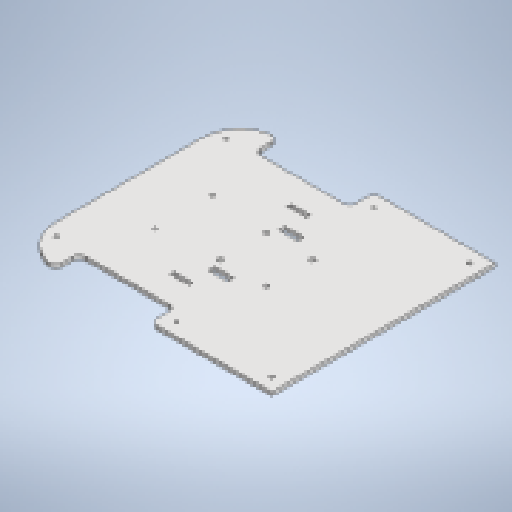
# Autodesk Inventor part: Base_Carro
Saved by Autodesk Inventor 2024 (Build 280153000, 153)
## iProperties
Created: 2025-05-13
Part Number: Base_Carro
Material: Genérico
Document SubType Name: Modeling
Designer: mario
Density: 1 g/cm^3
Appearance: Valor por defecto
Author: mario
Autodesk Inventor part; units mm, degrees
ref_plane "YZ Plane" through (0, 0, 0) normal (1, 0, 0) x (0, 1, 0)
ref_plane "XZ Plane" through (0, 0, 0) normal (0, 1, 0) x (-1, 0, 0)
ref_plane "XY Plane" through (0, 0, 0) normal (0, 0, 1) x (1, 0, 0)
sketch "Boceto1" plane through (0, 0, 0) normal (0, 1, 0) x (-1, 0, 0)
  line L0 (100, 87.5) -> (-100, 87.5)
  line L1 (-100, 87.5) -> (-100, -87.5)
  line L2 (-100, -87.5) -> (100, -87.5)
  line L3 (100, -87.5) -> (100, 87.5)
  line L4 (100, 87.5) -> (-100, -87.5) construction
  line L5 (-100, 87.5) -> (100, -87.5) construction
  point P0 (0, 0)
  dimension "d0" = 175
  dimension "d1" = 200
  constraints: 12 end point, 2 midpoint, 2 parallel, 1 horizontal, 1 perpendicular
  measures "d0" distance of L2.end L0.start
  measures "d1" distance of L1.end L2.end
extrude "Extrusión1" add sketch "Boceto1" along normal blind 3
sketch "Boceto2" plane through (0, 3, 0) normal (0, 1, 0) x (1, 0, 0)
  line L0 (-4.8, 47.5) -> (-20, 47.5)
  line L1 (-20, 47.5) -> (-20, 44.4)
  line L2 (-20, 44.4) -> (-4.8, 44.4)
  line L3 (-4.8, 44.4) -> (-4.8, 47.5)
  line L4 (100, 87.5) -> (-100, 87.5) construction
  line L5 (-100, 87.5) -> (-100, -87.5) construction
  point P0 (0, 0)
  dimension "d4" = 15.2
  dimension "d5" = 3.1
  dimension "d6" = 40
  dimension "d7" = 80
  constraints: 8 end point, 2 parallel, 1 horizontal, 1 perpendicular
  measures "d4" distance of L2.end L1.end
  measures "d5" distance of L2.end L0.start
  measures "d6" distance between parallel lines of L4 L0
  measures "d7" distance between parallel lines of L5 L1
extrude "Extrusión2" cut sketch "Boceto2" against normal blind 3
fillet "Empalme1" radius 30 2 edges at (-100, 1.5, -87.5) (-100, 1.5, 87.5)
sketch "Boceto3" plane through (0, 0, 0) normal (0, -1, 0) x (1, 0, 0)
  line L0 (-70, -87.5) -> (5, -87.5)
  line L1 (5, -87.5) -> (5, -68.5)
  line L2 (5, -68.5) -> (-70, -68.5)
  line L3 (-70, -68.5) -> (-70, -87.5)
  point P0 (0, 0)
  dimension "d11" = 75
  dimension "d12" = 19
  constraints: 8 end point, 2 parallel, 1 horizontal, 1 perpendicular
  measures "d11" distance of L1.end L2.end
  measures "d12" distance of L0.end L1.end
extrude "Extrusión3" cut sketch "Boceto3" against normal blind 3
mirror "Simetría1" about plane through (0, 0, 0) normal (0, 0, 1) of "Extrusión3"
fillet "Empalme3" radius 5 8 edges at (-70, 1.5, 87.5) (-70, 1.5, 68.5) (5, 1.5, 68.5) (5, 1.5, 87.5) (-70, 1.5, -87.5) (-70, 1.5, -68.5) (5, 1.5, -68.5) (5, 1.5, -87.5)
mirror "Simetría2" about plane through (0, 0, 0) normal (0, 0, 1) of "Extrusión2"
sketch "Boceto6" plane through (0, 3, 0) normal (0, 1, 0) x (1, 0, 0)
  line L0 (-100, 57.5) -> (-100, -57.5) construction
  line L1 (-10, -18.1) -> (26.2, -18.1) construction
  line L2 (-100, 0) -> (100, 0) construction
  line L3 (100, -87.5) -> (100, 87.5) construction
  line L4 (100, 87.5) -> (100, -87.5) construction
  point P0 (0, 0)
  point P1 (-10, 18.1)
  point P2 (26.2, 18.1)
  dimension "d36" = 90
  dimension "d37" = 36.2
  dimension "d38" = 36.2
  dimension "d39" = 18.1
  constraints: 6 end point, 4 symmetric about line, 2 horizontal, 2 midpoint
  measures "d36" distance from line of L0 L1.start
  measures "d37" distance of L1.end L1.start
  measures "d38" distance of point (-10, 18.1) L1.start
  measures "d39" distance from line of L1.start L2
hole "Agujero3" at (-10, 3, 18.1) at (26.2, 3, 18.1) at (-10, 3, -18.1) at (26.2, 3, -18.1) direction (0, -1, 0) diameter 4 end through all
sketch "Boceto7" plane through (0, 3, 0) normal (0, 1, 0) x (1, 0, 0)
  line L0 (-7.5, -30) -> (7.5, -30)
  line L1 (7.5, -30) -> (7.5, -25)
  line L2 (7.5, -25) -> (-7.5, -25)
  line L3 (-7.5, -25) -> (-7.5, -30)
  point P0 (0, 0)
  point P1 (0, -25)
  dimension "d47" = 5
  dimension "d48" = 15
  dimension "d49" = 25
  constraints: 8 end point, 2 parallel, 1 horizontal, 1 midpoint, 1 perpendicular, 1 vertical alignment
  measures "d47" distance of L2.end L0.start
  measures "d48" distance of L1.end L2.end
  measures "d49" distance from line of point (0, 0) L2
extrude "Extrusión4" cut sketch "Boceto7" against normal blind 3
mirror "Simetría3" about plane through (0, 0, 0) normal (0, 0, 1) of "Extrusión4"
sketch "Boceto9" plane through (0, 3, 0) normal (0, 1, 0) x (1, 0, 0)
  line L0 (-85, 22.7) -> (-85, -22.7) construction
  line L1 (100, -87.5) -> (100, 87.5) construction
  line L2 (100, 0) -> (-100, 0) construction
  line L3 (-56.552, 22.7) -> (-56.552, -22.7) construction
  line L4 (-100, 57.5) -> (-100, -57.5) construction
  point P0 (0, 0)
  point P1 (-85, 0)
  dimension "d52" = 28.448
  dimension "d54" = 45.4
  dimension "d55" = 15
  constraints: 6 end point, 3 midpoint, 2 coincident, 2 vertical, 1 horizontal, 1 horizontal alignment, 1 parallel, 1 point on line
  measures "d52" distance between parallel lines of L0 L3
  measures "d54" distance of L0.end L0.start
  measures "d55" distance between parallel lines of L4 L0
hole "Agujero4" at (-56.552, 3, -22.7) at (-56.552, 3, 22.7) direction (0, -1, 0) diameter 3 end through all
sketch "Boceto10" plane through (0, 3, 0) normal (0, 1, 0) x (1, 0, 0)
  line L0 (-65, -68.5) -> (0, -68.5) projected
  line L1 (-90, -66.5) -> (-90, 66.5) construction
  line L2 (-100, 57.5) -> (-100, -57.5) construction
  line L3 (90, -77.5) -> (15, -77.5) construction
  line L4 (90, 77.5) -> (15, 77.5) construction
  line L5 (100, -87.5) -> (100, 87.5) construction
  line L6 (5, 82.5) -> (5, 73.5) construction
  line L7 (100, 87.5) -> (10, 87.5) construction
  line L8 (10, -87.5) -> (100, -87.5) construction
  point P0 (0, 0)
  point P1 (-90, 0)
  dimension "d63" = 2
  dimension "d64" = 10
  dimension "d65" = 10
  dimension "d66" = 10
  dimension "d67" = 10
  dimension "d68" = 10
  constraints: 6 end point, 2 horizontal, 2 vertical alignment, 1 horizontal alignment, 1 midpoint, 1 parallel, 1 vertical
  measures "d63" distance from line of L0 L1.start
  measures "d64" distance between parallel lines of L2 L1
  measures "d65" distance from line of L5 L4.start
  measures "d66" distance from line of L6 L4.end
  measures "d67" distance between parallel lines of L7 L4
  measures "d68" distance between parallel lines of L8 L3
hole "Agujero5" at (90, 3, -77.5) at (15, 3, -77.5) at (90, 3, 77.5) at (15, 3, 77.5) at (-90, 3, -66.5) at (-90, 3, 66.5) direction (0, -1, 0) diameter 3 end through all
